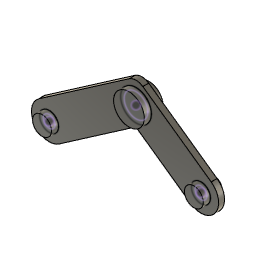
gd for rear leg base design (Autodesk Fusion 360 design; units mm, degrees)
Autodesk Fusion 360 part; units mm, degrees
sketch "Sketch1" plane through (0, 0, 0) normal (0, 1, 0) x (1, 0, 0)
  line L0 (40, -30) -> (116.4622, -82.9353)
  line L1 (127.9335, -82.8743) -> (185.8741, -41.8427)
  line L2 (57.0763, -5.3342) -> (122.0244, -50.2983)
  line L3 (122.0244, -50.2983) -> (168.5363, -17.3601)
  arc A0 (57.0763, -5.3342) -> (40, -30) centre (48.5381, -17.6671) ccw
  arc A1 (185.8741, -41.8427) -> (168.5363, -17.3601) centre (177.2052, -29.6014) ccw
  arc A2 (116.4622, -82.9353) -> (127.9335, -82.8743) centre (122.1543, -74.7134) ccw
  circle A3 centre (48.5381, -17.6671) radius 5
  circle A4 centre (177.2052, -29.6014) radius 5
  circle A5 centre (122.1543, -66.2983) radius 10
  point P0 (122.2192, -86.921)
  dimension "d1" = 100
  dimension "d2" = 78
  dimension "d3" = 110
  dimension "d4" = -30
  dimension "d5" = 10
  dimension "d6" = 10
  dimension "d7" = 10
  dimension "d8" = 20
  dimension "d9" = 16
  constraint coincident P0 L0
  constraint coincident P0 L1
  constraint tangent L0 A2
  constraint tangent L1 A2
  constraint concentric A0 A3
  constraint concentric A1 A4
  measures "d1" distance of L0.start P0
  measures "d2" distance of P0 L1.end
  measures "d3" angle of L0 L1
  measures "d5" radius of A2
  measures "d6" diameter of A3
  measures "d7" diameter of A4
  measures "d8" diameter of A5
  measures "d9" vertical distance of L2.end A5.centre
extrude "Extrude1" add sketch "Sketch1" along normal blind 5 makes body 1
sketch "Sketch1 (2)" plane through (0, 0, 0) normal (0, 1, 0) x (1, 0, 0) in component "preserve"
  circle A0 centre (122.1543, -66.2983) radius 10
  circle A1 centre (48.5381, -17.6671) radius 5
  circle A2 centre (177.2052, -29.6014) radius 5
  circle A3 centre (122.1543, -66.2983) radius 12
  circle A4 centre (177.2052, -29.6014) radius 7
  circle A5 centre (48.5381, -17.6671) radius 7
  dimension "d19" = 2
  dimension "d20" = 2
  dimension "d21" = 2
extrude "Extrude1'" add sketch "Sketch1 (2)" along normal blind 5 separate body makes body 2 at (134.1394, 3.3333, 66.8964) makes body 3 at (55.5294, 3.3333, 18.016) makes body 4 at (174.9758, 3.3333, 36.2369) in component "preserve"
sketch "Sketch1 (3)" plane through (0, 0, 0) normal (0, 1, 0) x (1, 0, 0) in component "obstacle"
  circle A0 centre (122.1543, -66.2983) radius 10
  circle A1 centre (48.5381, -17.6671) radius 5
  circle A2 centre (177.2052, -29.6014) radius 5
extrude "Extrude1''" add sketch "Sketch1 (3)" along normal blind 5 separate body makes body 5 at (132.1418, 3.3333, 66.7967) makes body 6 at (53.5319, 3.3333, 17.9163) makes body 7 at (182.199, 3.3333, 29.8506) in component "obstacle"
sketch "Sketch2" plane through (0, 0, 0) normal (0, -1, 0) x (1, 0, 0) in component "obstacle"
  circle A0 centre (122.1543, 66.2983) radius 10
  circle A1 centre (122.1543, 66.2983) radius 10
  circle A2 centre (48.5381, 17.6671) radius 5
  circle A3 centre (177.2052, 29.6014) radius 5
  circle A4 centre (122.1543, 66.2983) radius 13
  circle A5 centre (177.2052, 29.6014) radius 8
  circle A6 centre (48.5381, 17.6671) radius 8
  dimension "d26" = 3
  dimension "d27" = 3
  dimension "d28" = 3
extrude "Extrude2" add sketch "Sketch2" along normal blind 6 contours A0 A1 | A2 | A3 | A4 | A5 | A6 bodies 5 6 7 in component "obstacle"
sketch "Sketch3" plane through (0, 0, 0) normal (0, 1, 0) x (1, 0, 0) in component "obstacle"
  circle A0 centre (122.1543, -66.2983) radius 10
  circle A1 centre (177.2052, -29.6014) radius 5
  circle A2 centre (48.5381, -17.6671) radius 5
  circle A3 centre (122.1543, -66.2983) radius 13
  circle A4 centre (177.2052, -29.6014) radius 8
  circle A5 centre (48.5381, -17.6671) radius 8
  dimension "d31" = 3
  dimension "d32" = 3
  dimension "d33" = 3
extrude "Extrude3" add 3 faces at (133.4057, 5, 67.3913) (175.4627, 5, 35.6731) (54.8268, 5, 18.2633) along direction (0, 1, 0) blind 6 separate body on bodies 2 3 4 makes body 8 at (174.9758, 7, 36.2369) makes body 9 at (134.1394, 9, 66.8964) makes body 10 at (55.5294, 9, 18.016) in component "obstacle"
extrude "Extrude4" add 3 faces at (124.9084, 5, 68.176) (176.3254, 5, 27.3595) (49.5773, 5, 16.3641) along direction (0, 1, 0) blind 6 on bodies 5 6 7 bodies 5 6 7 8 9 10 in component "obstacle"
component "preserve" placed x (1, 0, 0) y (0, 1, 0) z (0, 0, 1) at (0, 0, 0)
component "obstacle" placed x (1, 0, 0) y (0, 1, 0) z (0, 0, 1) at (0, 0, 0)
